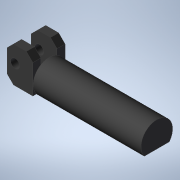
# Autodesk Inventor part: Hammer
Saved by Autodesk Inventor 2021 (Build 250183000, 183)
## iProperties
Created: 2021-03-07
Part Number: Hammer
Material: Generic
Document SubType Name: Modeling
Designer: Lukas
Density: 1 g/cm^3
Appearance: Default
Author: Lukas
Autodesk Inventor part; units mm, degrees
ref_plane "YZ Plane" through (0, 0, 0) normal (1, 0, 0) x (0, 1, 0)
ref_plane "XZ Plane" through (0, 0, 0) normal (0, 1, 0) x (-1, 0, 0)
sketch "Sketch5" plane through (0, 0, 0) normal (0, 0, 1) x (1, 0, 0)
  line L0 (-33.5, 0) -> (0, 0)
  line L1 (0, 4.9) -> (0, 0)
  line L2 (-33.5, 4.9) -> (0, 4.9)
  line L3 (-33.5, 4.9) -> (-33.5, 0)
  dimension "d95" = 4.9
  dimension "d106" = 33.5
  constraints: 8 end point, 2 horizontal, 2 vertical
  measures "d95" distance of L1.start L0.end
  measures "d106" distance of L2.start L1.start
revolve "Revolution1" add sketch "Sketch5" angle 360 about axis through (-33.5, 0, 0) along (1, 0, 0)
sketch "Sketch6" plane through (0, 0, 0) normal (1, 0, 0) x (0, 0, -1)
  circle A0 centre (0, 0) radius 4.9 projected
  circle A1 centre (0, 0) radius 4.9 projected
  line L0 (-3.8743, -3) -> (3.8743, -3)
  dimension "d96" = 3
  constraints: 2 end point, 2 point on circle, 1 horizontal
  measures "d96" distance from line of point (0, 0) L0
extrude "Extrusion5" cut sketch "Sketch6" against normal blind 53 contours L0 A0 picked at (-1.032, -3.266)
ref_plane "Work Plane2" through (0, 0, -2.5) normal (0, 0, 1) x (1, 0, 0)
sketch "Sketch10" plane through (0, 0, -2.5) normal (0, 0, 1) x (1, 0, 0)
  line L0 (-33.5, -3) -> (-33.5, -3) projected
  line L1 (-33.5, -3) -> (-33.5, 4.9) projected
  line L2 (-33.5, -3) -> (-39.5, -3)
  line L3 (-39.5, -3) -> (-41.5, -1)
  line L4 (-41.5, -1) -> (-41.5, 6)
  line L5 (-41.5, 6) -> (-39.5, 8)
  line L6 (-39.5, 8) -> (-35.5, 8)
  line L7 (-35.5, 8) -> (-33.5, 6)
  line L8 (-33.5, 6) -> (-33.5, 4.9)
  circle A0 centre (-39, 3) radius 1.4
  point P0 (0, 0)
  dimension "d127" = 45
  dimension "d128" = 2
  dimension "d129" = 6
  dimension "d130" = 2
  dimension "d131" = 7
  dimension "d132" = 2.8
  dimension "d133" = 5
  dimension "d136" = 2.5
  constraints: 14 end point, 4 perpendicular, 1 centre point, 1 collinear, 1 horizontal, 1 parallel
  measures "d127" angle of L2 L3
  measures "d128" horizontal distance of L2.end L3.end
  measures "d129" distance of L0.end L2.end
  measures "d130" horizontal distance of L4.end L5.end
  measures "d131" distance of L3.end L4.end
  measures "d132" diameter of A0
  measures "d133" distance from line of L6 A0.centre
  measures "d136" distance from line of L4 A0.centre
extrude "Extrusion9" add sketch "Sketch10" against normal blind 2.5
mirror "Mirror1" about plane through (0, 0, 0) normal (0, 0, 1) of "Extrusion9"
chamfer "Chamfer3" distance 4.5 distance2 2.5 1 edges at (-33.5, -3, 0) measured on face at (-33.5, -2.5, 0)
body "Solid2"
